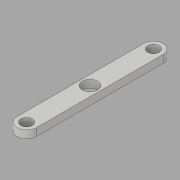
# Autodesk Inventor part: g_servo horn
Saved by Autodesk Inventor 2019 (Build 230136000, 136)
## iProperties
Created: 2021-10-30
Part Number: g_servo horn
Material: Generic
Document SubType Name: Modeling
Designer: Mohamed
Density: 1 g/cm^3
Appearance: Default
Author: Mohamed
Autodesk Inventor part; units mm, degrees
ref_plane "YZ Plane" through (0, 0, 0) normal (1, 0, 0) x (0, 1, 0)
ref_plane "XZ Plane" through (0, 0, 0) normal (0, 1, 0) x (-1, 0, 0)
ref_plane "XY Plane" through (0, 0, 0) normal (0, 0, 1) x (1, 0, 0)
sketch "Sketch1" plane through (0, 0, 0) normal (0, 1, 0) x (-1, 0, 0)
  arc A0 (2.5, 0) -> (-2.5, 0) centre (0, 0) ccw
  line L0 (2.5, 0) -> (2.5, -33)
  line L1 (-2.5, 0) -> (-2.5, -33)
  arc A1 (-2.5, -33) -> (2.5, -33) centre (0, -33) ccw
  circle A2 centre (0, -16.5) radius 2
  circle A3 centre (0, 0) radius 1.5
  circle A4 centre (0, -33) radius 1.5
  dimension "d11" = 5
  dimension "d12" = 33
  dimension "d13" = 33
  dimension "d14" = 5
  dimension "d15" = 4
  dimension "d16" = 3
  dimension "d17" = 3
  constraints: 5 centre point, 4 end point, 4 point on circle, 2 coincident, 2 vertical, 1 tangent
  measures "d11" diameter of A0
  measures "d12" distance of L0.start L0.end
  measures "d13" distance of L1.start L1.end
  measures "d14" diameter of A1
  measures "d15" diameter of A2
  measures "d16" diameter of A3
  measures "d17" diameter of A4
extrude "Extrusion1" add sketch "Sketch1" along normal blind 2
body "Solid1"
